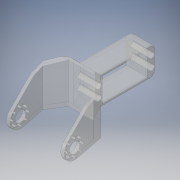
# Autodesk Inventor part: Femur
Saved by Autodesk Inventor 2016 (Build 200138000, 138)
## iProperties
Created: 2016-05-19
Part Number: Femur
Material: PET Plastic
Document SubType Name: Modeling
Designer: kromm.je.s
Density: 1.541 g/cm^3
Appearance: Polycarbonate - Smoked
Mass: 38.9251 g
Surface Area: 159.101 cm^2
Volume: 25.2597 cm^3
Author: kromm.je.s
Autodesk Inventor part; units mm, degrees
ref_plane "YZ Plane" through (0, 0, 0) normal (1, 0, 0) x (0, 1, 0)
ref_plane "XZ Plane" through (0, 0, 0) normal (0, 1, 0) x (-1, 0, 0)
ref_plane "XY Plane" through (0, 0, 0) normal (0, 0, 1) x (1, 0, 0)
sketch "Sketch1" plane through (0, 0, 0) normal (0, 1, 0) x (-1, 0, 0)
  line L0 (-10.5, 20.5) -> (10.5, 20.5)
  line L1 (10.5, 20.5) -> (10.5, -20.5)
  line L2 (10.5, -20.5) -> (-10.5, -20.5)
  line L3 (-10.5, -20.5) -> (-10.5, 20.5)
  line L4 (-10.5, 20.5) -> (10.5, -20.5) construction
  line L5 (10.5, 20.5) -> (-10.5, -20.5) construction
  line L6 (-13.5, 28.5) -> (13.5, 28.5)
  line L7 (13.5, 28.5) -> (13.5, -28.5)
  line L8 (13.5, -28.5) -> (-13.5, -28.5)
  line L9 (-13.5, -28.5) -> (-13.5, 28.5)
  line L10 (-13.5, 28.5) -> (13.5, -28.5) construction
  line L11 (13.5, 28.5) -> (-13.5, -28.5) construction
  point P0 (0, 0)
  point P1 (0, 0)
  dimension "d0" = 21
  dimension "d1" = 41
  dimension "d2" = 27
  dimension "d3" = 57
  constraints: 24 end point, 6 midpoint, 4 parallel, 2 horizontal, 2 perpendicular
  measures "d0" distance of L1.end L2.end
  measures "d1" distance of L0.end L1.end
  measures "d2" distance of L7.end L8.end
  measures "d3" distance of L6.end L7.end
extrude "Extrusion1" add sketch "Sketch1" along normal blind 20
sketch "Sketch2" plane through (0, 20, 0) normal (0, 1, 0) x (1, 0, 0)
  line L0 (-10.5, -20.5) -> (-10.5, 20.5) projected
  line L1 (-10.5, 20.5) -> (10.5, 20.5) projected
  line L2 (10.5, 20.5) -> (10.5, -20.5) projected
  line L3 (10.5, -20.5) -> (-10.5, -20.5) projected
  line L4 (-13.5, -28.5) -> (13.5, -28.5) projected
  line L5 (13.5, -28.5) -> (13.5, 28.5) projected
  line L6 (13.5, 28.5) -> (-13.5, 28.5) projected
  line L7 (-13.5, 28.5) -> (-13.5, -28.5) projected
  line L8 (10.5, -20.5) -> (-10.5, -20.5) projected
  line L9 (0, -20.5) -> (0, -25)
  line L10 (0, -25) -> (-5, -25)
  line L11 (0, -25) -> (5, -25)
  line L12 (0, 20.5) -> (0, 25)
  line L13 (0, 25) -> (-5, 25)
  line L14 (0, 25) -> (5, 25)
  circle A0 centre (-5, -25) radius 2.5
  circle A1 centre (5, -25) radius 2.5
  circle A2 centre (-5, 25) radius 2.5
  circle A3 centre (5, 25) radius 2.5
  point P0 (0, 0)
  dimension "d6" = 4.5
  dimension "d7" = 5
  dimension "d8" = 5
  dimension "d9" = 4.5
  dimension "d10" = 5
  dimension "d11" = 5
  dimension "d12" = 5
  dimension "d13" = 5
  dimension "d14" = 5
  dimension "d15" = 5
  constraints: 12 end point, 4 centre point, 4 coincident, 2 horizontal, 2 midpoint, 2 perpendicular, 2 vertical
  measures "d6" distance of L9.start L9.end
  measures "d7" distance of L9.end L10.end
  measures "d8" distance of L9.end L11.end
  measures "d9" distance of L12.start L12.end
  measures "d10" distance of L12.end L13.end
  measures "d11" distance of L12.end L14.end
  measures "d12" diameter of A0
  measures "d13" diameter of A1
  measures "d14" diameter of A2
  measures "d15" diameter of A3
extrude "Extrusion2" cut sketch "Sketch2" against normal blind 20 contours A0 | A1 | A2 | A3
sketch "Sketch3" plane through (-13.5, 0, 28.5) normal (0, 0, 1) x (1, 0, 0)
  line L0 (27, 0) -> (0, 0) projected
  line L1 (27, 0) -> (27, 20) projected
  line L2 (0, 20) -> (27, 20) projected
  line L3 (0, 0) -> (0, 20) projected
  line L4 (24, 20) -> (3, 20) projected
  line L5 (13.5, 20) -> (13.5, 0)
  line L6 (40.5, 37) -> (-13.5, 37)
  line L7 (-13.5, 37) -> (-13.5, -17)
  line L8 (-13.5, -17) -> (40.5, -17)
  line L9 (40.5, -17) -> (40.5, 37)
  line L10 (40.5, 37) -> (-13.5, -17) construction
  line L11 (-13.5, 37) -> (40.5, -17) construction
  point P0 (13.5, 10)
  dimension "d18" = 54
  dimension "d19" = 54
  constraints: 14 end point, 4 midpoint, 2 parallel, 1 horizontal, 1 perpendicular, 1 vertical
  measures "d18" distance of L8.end L7.end
  measures "d19" distance of L7.end L6.end
extrude "Extrusion3" add sketch "Sketch3" along normal blind 46 contours L0 L5 L2 L1 | L0 L3 L2 L5 | L9 L8 L7 L6
sketch "Sketch4" plane through (-27, 37, 28.5) normal (0, 1, 0) x (1, 0, 0)
  line L0 (54, 0) -> (0, 0) projected
  line L1 (0, 0) -> (0, -46) projected
  line L2 (54, -46) -> (0, -46) projected
  line L3 (54, 0) -> (54, -46) projected
  line L4 (40.5, 0) -> (40.5, 57) projected
  line L5 (40.5, 0) -> (45.5, 0)
  line L6 (0, 0) -> (54, 0) projected
  line L7 (45.5, 0) -> (45.5, -15)
  line L8 (13.5, 0) -> (13.5, 57) projected
  line L9 (13.5, 0) -> (8.5, 0)
  line L10 (54, -46) -> (0, -46) projected
  line L11 (0, -46) -> (0, -36)
  line L12 (0, 0) -> (0, -46) projected
  line L13 (0, -36) -> (10, -36)
  circle A0 centre (10, -36) radius 10
  line L14 (45.5, -15) -> (17.0262, -43.1157)
  line L15 (8.5, 0) -> (0.2856, -33.627)
  line L16 (40.5, 0) -> (54, 20.4237)
  line L17 (54, 20.4237) -> (69.128, 3.8924)
  line L18 (69.128, 3.8924) -> (67.0453, -50.908)
  line L19 (67.0453, -50.908) -> (51.4859, -70.7132)
  line L20 (51.4859, -70.7132) -> (6.3874, -70.7132)
  line L21 (6.3874, -70.7132) -> (-10.1482, -68.6543)
  line L22 (-10.1482, -68.6543) -> (-23.5511, -46.3521)
  line L23 (-23.5511, -46.3521) -> (-23.5511, -25.0047)
  line L24 (-23.5511, -25.0047) -> (-16.8497, -1.0127)
  line L25 (-16.8497, -1.0127) -> (-4.584, 10.2118)
  line L26 (-4.584, 10.2118) -> (13.5, 0)
  point P0 (27, 28.5)
  dimension "d22" = 5
  dimension "d23" = 15
  dimension "d24" = 5
  dimension "d26" = 10
  dimension "d27" = 10
  dimension "d28" = 20
  constraints: 36 end point, 3 perpendicular, 3 point on line, 2 horizontal, 2 point on circle, 2 tangent, 1 centre point, 1 coincident
  measures "d22" distance of L4.start L5.end
  measures "d23" distance of L5.end L7.end
  measures "d24" distance of L8.start L9.end
  measures "d26" distance of L1.end L11.end
  measures "d27" distance of L11.end L13.end
  measures "d28" diameter of A0
extrude "Extrusion4" cut sketch "Sketch4" against normal blind 75.25 contours L3 L2 A0 L14 L7 L0 | L0 L16 L17 L18 L19 L20 L21 L22 L23 L24 L25 L26 L1 L2 L3 | L2 L1 A0 | L1 L0 L15 A0
sketch "Sketch5" plane through (18.5, 37, 43.5) normal (1, 0, 0) x (0, 0, -1)
  line L0 (15, -54) -> (0, -54) projected
  line L1 (15, 0) -> (15, -54) projected
  line L2 (0, 0) -> (15, 0) projected
  line L3 (0, 0) -> (0, -54) projected
  line L4 (0, -54) -> (-28.1157, -54) projected
  line L5 (0, 0) -> (0, -54) projected
  line L6 (-28.1157, 0) -> (0, 0) projected
  line L7 (-28.1157, 0) -> (-28.1157, -54) projected
  line L8 (-28.1157, -54) -> (-18.627, -54) projected
  line L9 (-28.1157, 0) -> (-28.1157, -54) projected
  line L10 (-18.627, 0) -> (-28.1157, 0) projected
  line L11 (-18.627, 0) -> (-18.627, -54) projected
  line L12 (-31, -54) -> (-31, 0) projected
  line L13 (15, -54) -> (12, -54)
  line L14 (15, -54) -> (0, -54) projected
  line L15 (15, 0) -> (15, -54) projected
  line L16 (15, 0) -> (12, 0)
  line L17 (0, 0) -> (15, 0) projected
  line L18 (12, -54) -> (12, -51)
  line L19 (12, 0) -> (12, -3)
  line L20 (12, -51) -> (-31, -51)
  line L21 (-31, -51) -> (-31, -3)
  line L22 (-31, -3) -> (12, -3)
  line L23 (12, -3) -> (12, -51)
  point P0 (43.5, -37)
  dimension "d31" = 3
  dimension "d32" = 3
  dimension "d33" = 3
  dimension "d34" = 3
  constraints: 16 end point, 3 point on line, 2 parallel, 2 vertical, 1 horizontal, 1 perpendicular
  measures "d31" distance of L0.start L13.end
  measures "d32" distance of L1.start L16.end
  measures "d33" distance of L13.end L18.end
  measures "d34" distance of L16.end L19.end
extrude "Extrusion5" cut sketch "Sketch5" against normal blind 75.25 contours L20 L3 L22 L23 | L20 L11 L22 L3 | L20 L7 L22 L11 | L20 L12 L22 L7
sketch "Sketch6" plane through (-18.5, 37, 28.5) normal (0, 1, 0) x (1, 0, 0)
  line L0 (0, 0) -> (-8.2144, -33.627) projected
  arc A0 (-8.2144, -33.627) -> (8.5262, -43.1157) centre (1.5, -36) ccw projected
  line L1 (8.5262, -43.1157) -> (37, -15) projected
  line L2 (37, -15) -> (37, 0) projected
  line L3 (37, 0) -> (0, 0) projected
  circle A1 centre (1.5, -36) radius 5
  point P0 (18.5, 28.5)
  dimension "d37" = 10
  constraints: 1 centre point, 1 coincident
  measures "d37" diameter of A1
extrude "Extrusion6" cut sketch "Sketch6" against normal blind 75.25 contours A1
fillet "Fillet1" radius 5 2 edges at (13.5, 10, -28.5) (-13.5, 10, -28.5)
chamfer "Chamfer1" distance 5 angle 45 2 edges at (13.5, 10, 28.5) (-13.5, 10, 28.5)
chamfer "Chamfer2" distance 12 angle 45 2 edges at (-0.3664, 34, 31.5) (-0.3664, -14, 31.5)
chamfer "Chamfer3" distance 12 angle 45 2 edges at (0, 37, 28.5) (0, -17, 28.5)
sketch "Sketch7" plane through (-21.4313, 37, 40.5) normal (0, 1, 0) x (1, 0, 0)
  line L0 (0, 0) -> (39.9313, 0) projected
  line L1 (0, 0) -> (-5.283, -21.627) projected
  arc A0 (-5.283, -21.627) -> (11.4575, -31.1157) centre (4.4313, -24) ccw projected
  line L2 (11.4575, -31.1157) -> (39.9313, -3) projected
  line L3 (39.9313, -3) -> (39.9313, 0) projected
  circle A1 centre (4.4313, -24) radius 5 projected
  circle A2 centre (4.4313, -24) radius 7.5
  circle A3 centre (4.4313, -31.5) radius 0.75
  point P0 (21.4313, 40.5)
  dimension "d50" = 15
  dimension "d51" = 1.5
  constraints: 1 centre point, 1 coincident, 1 vertical alignment, 2 other
  measures "d51" diameter of A3
extrude "Extrusion7" cut sketch "Sketch7" against normal blind 70 contours A3 A2 | A2 A3 picked at (4.4021, -31.2489) picked at (4.4557, -31.746)
pattern_circular "Circular Pattern1" count 8 over 360 about axis through (-17, 37, 64.5) along (0, -1, 0) of "Extrusion7"
fillet "Fillet2" radius 1 18 edges at (10.5, 20, 0) (0, 20, 20.5) (-10.5, 20, 0) (-10.5, 0, 0) (0, 0, 20.5) (10.5, 0, 0) (0, 20, -20.5) (0, 0, -20.5) (-12.0355, 20, -27.0355) (0, 20, -28.5) (12.0355, 20, -27.0355) (13.5, 20, 0.0001) (-13.5, 20, 0.0001) (-12.0355, 0, -27.0355) (0, 0, -28.5) (12.0355, 0, -27.0355) (13.5, 0, 0.0001) (-13.5, 0, 0.0001)
chamfer "Chamfer4" distance 12 angle 45 2 edges at (18.5, 35.5, 43.5) (18.5, -15.5, 43.5)
body "Solid1"
